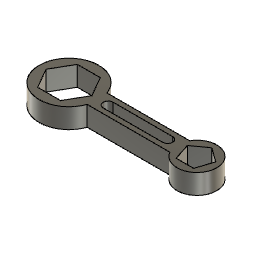
Exercise _02 (Autodesk Fusion 360 design; units mm, degrees)
Autodesk Fusion 360 part; units mm, degrees
sketch "Sketch1" plane through (0, 0, 0) normal (0, 1, 0) x (1, 0, 0)
  line L0 (64.5, 10) -> (-64.5, 10)
  line L1 (-64.5, 10) -> (-64.5, -10)
  line L2 (-64.5, -10) -> (64.5, -10)
  line L3 (64.5, -10) -> (64.5, 10)
  line L4 (64.5, 10) -> (-64.5, -10) construction
  line L5 (-64.5, 10) -> (64.5, -10) construction
  line L6 (35, 0) -> (39.5, 0) construction
  line L7 (-35, 0) -> (-39.5, 0) construction
  circle A0 centre (-69.5, 0) radius 30
  circle A1 centre (59.5, 0) radius 20
  line L8 (59.5, 0) -> (59.5, 15) construction
  line L9 (-69.5, 0) -> (-69.5, 20) construction
  line L10 (-81.047, 20) -> (-92.594, 0)
  line L11 (-92.594, 0) -> (-81.047, -20)
  line L12 (-81.047, -20) -> (-57.953, -20)
  line L13 (-57.953, -20) -> (-46.406, 0)
  line L14 (-46.406, 0) -> (-57.953, 20)
  line L15 (-57.953, 20) -> (-81.047, 20)
  line L16 (59.5, 0) -> (59.5, -15) construction
  line L17 (50.6832, 12.1353) -> (45.2341, -4.6353)
  line L18 (45.2341, -4.6353) -> (59.5, -15)
  line L19 (59.5, -15) -> (73.7659, -4.6353)
  line L20 (73.7659, -4.6353) -> (68.3168, 12.1353)
  line L21 (68.3168, 12.1353) -> (50.6832, 12.1353)
  line L22 (35, 5) -> (-35, 5)
  line L23 (-35, 5) -> (-35, -5)
  line L24 (-35, -5) -> (35, -5)
  line L25 (35, -5) -> (35, 5)
  line L26 (35, 5) -> (-35, -5) construction
  line L27 (-35, 5) -> (35, -5) construction
  circle A2 centre (30, 0) radius 5
  circle A3 centre (-30, 0) radius 5
  point P0 (-35, 5)
  point P1 (-35, -5)
  point P2 (59.5, 0)
  point P3 (-69.5, 0)
  point P4 (59.5, 0)
  dimension "d2" = 10
  dimension "d4" = 129
  dimension "d5" = 20
  dimension "d6" = 4.5
  dimension "d7" = 4.5
  dimension "d8" = 60
  dimension "d9" = 40
  dimension "d10" = 15
  dimension "d11" = 20
  dimension "d12" = 15
  dimension "d13" = 12.1353
  dimension "d14" = 10
  dimension "d15" = 10
  dimension "d16" = 10
  constraint horizontal L0
  constraint perpendicular L0 L1
  constraint parallel L0 L2
  constraint parallel L1 L3
  constraint coincident L4 origin
  constraint coincident L5 origin
  constraint coincident P4 P2
  constraint perpendicular L0 L8
  constraint coincident P3 A0.centre
  constraint vertical L9
  constraint parallel L8 L16
  constraint horizontal L22
  constraint perpendicular L22 L23
  constraint parallel L22 L24
  constraint parallel L23 L25
  constraint coincident L26 origin
  constraint coincident L27 origin
  measures "d2" distance of P0 L23.end
  measures "d4" distance of L1.end L2.end
  measures "d5" distance of L0.end L1.end
  measures "d6" distance of L6.start L6.end
  measures "d7" distance of L7.start L7.end
  measures "d8" diameter of A0
  measures "d9" diameter of A1
  measures "d10" distance of P4 L8.end
  measures "d11" distance of P3 L9.end
  measures "d12" distance of P4 L16.end
  measures "d13" distance of P4 L21
  measures "d14" distance of P0 P1
  measures "d15" diameter of A2
  measures "d16" diameter of A3
extrude "Extrude1" add sketch "Sketch1" along normal mid plane 20 contours L0 L2 A1 L17 L18 | L0 L2 A1 L17 L18 L19 L20 L21 | L0 L2 A0 A1 | L0 L2 A0 L13 L14 | L0 L2 A0 L10 L11 L12 L13 L14 L15 | L22 L25 A2 | L24 L25 A2 | L22 L23 A3 | L23 L24 A3
move_body "Move1" bodies 1 to x (1, 0, 0) y (0, 0, -1) z (0, 1, 0) at (0, 5, 10)
